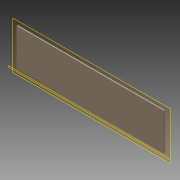
# Autodesk Inventor part: Panel_back
Saved by Autodesk Inventor 2013 (Build 170138000, 138)
## iProperties
Created: 2013-02-01
Part Number: Panel_back
Material: Aluminum 6061
Document SubType Name: Modeling
Designer: xylzlyx
Density: 1 g/cm^3
Author: xylzlyx
Autodesk Inventor part; units mm, degrees
ref_plane "YZ Plane" through (0, 0, 0) normal (1, 0, 0) x (0, 1, 0)
ref_plane "XZ Plane" through (0, 0, 0) normal (0, 1, 0) x (-1, 0, 0)
ref_plane "XY Plane" through (0, 0, 0) normal (0, 0, 1) x (1, 0, 0)
ref_plane "RecessedBackPanel" through (0, 0, -4) normal (0, 0, 1) x (1, 0, 0)
ref_plane "Work Plane1" through (0, 0, 0) normal (0, 0, 1) x (1, 0, 0)
sketch "Sketch1" plane through (0, 0, -4) normal (0, 0, 1) x (1, 0, 0)
  line L0 (0, 100.3251) -> (0, 97.2788) construction
  line L1 (0, 97.2788) -> (-375, 97.2788) construction
  line L2 (-375, 97.2788) -> (-375, 100.3251) construction
  line L3 (-375, 100.3251) -> (0, 100.3251) construction
  line L4 (0, -3) -> (-375, -3) construction
  line L5 (-375, -3) -> (-375, 0) construction
  line L6 (-375, 0) -> (0, 0) construction
  line L7 (0, 0) -> (0, -3) construction
  line L8 (-375, 94.2788) -> (0, 94.2788)
  line L9 (0, 94.2788) -> (0, 0)
  line L10 (0, 0) -> (-375, 0)
  line L11 (-375, 0) -> (-375, 94.2788)
  dimension "d4" = 3
  constraints: 24 end point, 5 horizontal, 4 vertical, 2 parallel, 2 vertical alignment, 1 coincident, 1 perpendicular, 7 other
  measures "d4" distance between parallel lines of L1 L8
extrude "Extrusion1" add sketch "Sketch1" against normal blind 3
fillet "Corners" radius 1 4 edges at (0, 94.2788, -5.5) (0, 0, -5.5) (-375, 94.2788, -5.5) (-375, 0, -5.5)
body "Solid1"
